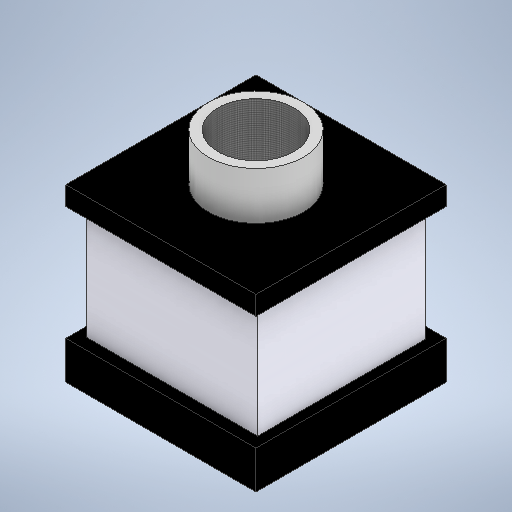
# Autodesk Inventor part: Camara
Saved by Autodesk Inventor 2025.2 (Build 292293000, 293)
## iProperties
Created: 2025-02-05
Part Number: Camara
Material: Generic
Document SubType Name: Modeling
Designer: Proyectos
Density: 1 g/cm^3
Appearance: Default
Author: Proyectos
Autodesk Inventor part; units mm, degrees
ref_plane "YZ Plane" through (0, 0, 0) normal (1, 0, 0) x (0, 1, 0)
ref_plane "XZ Plane" through (0, 0, 0) normal (0, 1, 0) x (-1, 0, 0)
ref_plane "XY Plane" through (0, 0, 0) normal (0, 0, 1) x (1, 0, 0)
sketch "Sketch1" plane through (0, 0, 0) normal (0, 1, 0) x (-1, 0, 0)
  line L0 (0, 0) -> (200, 0)
  line L1 (200, 0) -> (200, -200)
  line L2 (200, -200) -> (0, -200)
  line L3 (0, -200) -> (0, 0)
  dimension "d0" = 200
  dimension "d1" = 200
  constraints: 8 end point, 2 parallel, 1 horizontal, 1 perpendicular
  measures "d0" distance of L1.end L2.end
  measures "d1" distance of L2.end L0.start
extrude "Extrusion1" add sketch "Sketch1" along normal blind 40
sketch "Sketch2" plane through (0, 40, 0) normal (0, 1, 0) x (1, 0, 0)
  line L0 (0, 200) -> (-200, 200) projected
  line L1 (-200, 200) -> (-200, 0) projected
  line L2 (-200, 0) -> (0, 0) projected
  line L3 (0, 0) -> (0, 200) projected
  line L4 (-10, 11.7093) -> (-190, 11.7093)
  line L5 (-190, 11.7093) -> (-190, 188.2907)
  line L6 (-190, 188.2907) -> (-10, 188.2907)
  line L7 (-10, 188.2907) -> (-10, 11.7093)
  line L8 (-10, 11.7093) -> (-190, 188.2907) construction
  line L9 (-190, 11.7093) -> (-10, 188.2907) construction
  point P0 (-100, 100)
  dimension "d4" = 180
  constraints: 12 end point, 2 midpoint, 2 parallel, 1 horizontal, 1 perpendicular
  measures "d4" distance of L5.end L6.end
extrude "Extrusion2" add sketch "Sketch2" along normal blind 120 contours L4 L5 L6 L7
sketch "Sketch3" plane through (0, 160, 0) normal (0, 1, 0) x (1, 0, 0)
  line L0 (-10, 188.2907) -> (-190, 188.2907) projected
  line L1 (-190, 188.2907) -> (-190, 11.7093) projected
  line L2 (-190, 11.7093) -> (-10, 11.7093) projected
  line L3 (-10, 11.7093) -> (-10, 188.2907) projected
  line L4 (0, 0) -> (0, 200) projected
  line L5 (0, 200) -> (-200, 200) projected
  line L6 (0, 0) -> (-200, 0)
  line L7 (-200, 0) -> (-200, 200)
  line L8 (-200, 200) -> (0, 200)
  line L9 (0, 200) -> (0, 0)
  constraints: 8 end point, 2 parallel, 1 horizontal, 1 perpendicular
extrude "Extrusion3" add sketch "Sketch3" along normal blind 20 contours L3 L2 L1 L0 | L6 L7 L5 L4
sketch "Sketch4" plane through (0, 180, 0) normal (0, 1, 0) x (1, 0, 0)
  line L0 (-200, 200) -> (-200, 0) projected
  line L1 (-200, 200) -> (0, 0)
  line L2 (0, 200) -> (-200, 200) projected
  line L3 (-200, 0) -> (0, 200)
  circle A0 centre (-100, 100) radius 50
  dimension "d9" = 100
  constraints: 4 end point, 1 centre point, 1 midpoint
  measures "d9" diameter of A0
extrude "Extrusion4" add sketch "Sketch4" along normal blind 50 contours A0 L3 L1 | L1 L3 A0 | L3 L1 A0 | L3 A0 L1
sketch "Sketch5" plane through (-100, 230, -100) normal (0, 1, 0) x (1, 0, 0)
  circle A0 centre (0, 0) radius 40
  point P0 (100, -100)
  dimension "d12" = 80
  constraints: 1 centre point
  measures "d12" diameter of A0
extrude "Extrusion5" cut sketch "Sketch5" against normal blind 80
body "Solid1"
